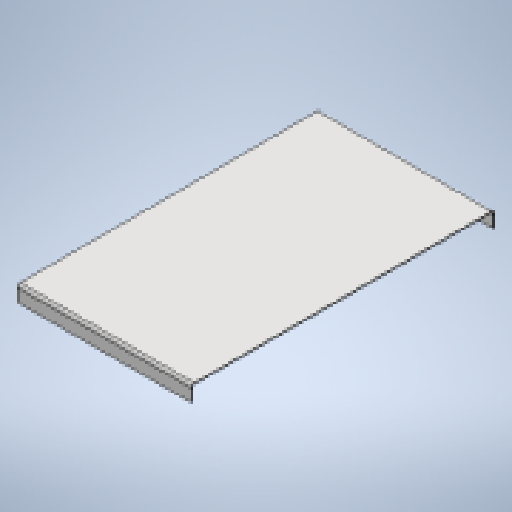
# Autodesk Inventor part: TRM 025 left board damper
Saved by Autodesk Inventor 2025 (Build 290162010, 162A)
## iProperties
Created: 2024-08-07
Part Number: TRM 025 left board damper
Material: AISI 304
Document SubType Name: Sheet Metal
Designer: pokla
Density: 8.02768 g/cm^3
Flat Pattern Width: 29 cm
Flat Pattern Length: 53.0404 cm
Flat Pattern Area: 1538.17 cm^2
Sheet Metal Rule: AISI304 2mm Die16
Sheet Metal Width: 290,000 mm
Sheet Metal Length: 530,404 mm
Sheet Metal Area: 153817,155 mm^2
Appearance: Default
Stock Number: ТРМ 025 левый борт успокоитель
Author: pokla
Autodesk Inventor part; units mm, degrees
ref_plane "YZ Plane" through (0, 0, 0) normal (1, 0, 0) x (0, 1, 0)
ref_plane "XZ Plane" through (0, 0, 0) normal (0, 1, 0) x (-1, 0, 0)
ref_plane "XY Plane" through (0, 0, 0) normal (0, 0, 1) x (1, 0, 0)
sketch "Sketch1" plane through (0, 0, 0) normal (0, 0, 1) x (1, 0, 0)
  line L0 (-145, -242) -> (145, -242)
  line L1 (145, -242) -> (145, 242)
  line L2 (145, 242) -> (-145, 242)
  line L3 (-145, 242) -> (-145, -242)
  line L4 (-145, -242) -> (145, 242) construction
  line L5 (145, -242) -> (-145, 242) construction
  point P0 (0, 0)
  dimension "d0" = 290
  dimension "d1" = 484
  measures "d0" distance of L2.end L1.end
  measures "d1" distance of L1.end L0.end
extrude "Plate1" add sketch "Sketch1" along normal blind 2
sketch "Sketch2" plane through (0, 0, 0) normal (0, 0, -1) x (-1, 0, 0)
  line L0 (-125, 222) -> (75, 222) construction
  line L1 (75, 222) -> (75, 202) construction
  line L2 (75, 202) -> (-125, 202) construction
  line L3 (-125, 202) -> (-125, 222) construction
  line L4 (-145, 242) -> (145, 242) projected
  line L5 (-145, -242) -> (-145, 242) projected
  point P0 (0, 0)
  point P1 (-48, 100)
  point P2 (-50, 98)
  dimension "d6" = 200
  dimension "d9" = 20
  dimension "d10" = 20
  dimension "d11" = 20
  constraints: 4 other
  measures "d6" distance of L0.start L0.end
  measures "d9" distance of L0.end L1.end
  measures "d11" length of L3
mark "Mark1"
sketch "Sketch3" plane through (-145, 244, 2) normal (0, -1, 0) x (1, 0, 0)
  line L0 (290, 0) -> (0, 0)
  line L1 (0, 0) -> (0, 25)
  line L2 (0, 25) -> (290, 25)
  line L3 (290, 25) -> (290, 0)
  constraints: 8 end point
edge flange "Flange1" height 25 angle 90 thickness 2 bend radius 2.75 thickness toward (0, -1, 0) relief round relief width 2 relief depth 1 corner gap 2.75 corner form 0 edges at (0, 242, 2) (0, -242, 2) wall of the first edge with corners at (145, 244, 2) (-145, 244, 2) (-145, 244, -23) (145, 244, -23)
bend "Bend1"
corner "Corner1"
equation "\"d2\" = Thickness"
equation "\"d12\" = BendReliefWidth"
equation "\"d13\" = BendReliefDepth"
equation "\"d14\" = MinimumRemnant"
equation "\"d15\" = TransitionRadius"
equation "\"d18\" = BendRadius"
equation "\"d19\" = CornerReliefSize"
equation "\"d20\" = GapSize"
equation "\"d21\" = JacobiRadiusSize"
equation "\"BendReliefWidth\" = Thickness"
equation "\"BendReliefDepth\" = 0.5 * Thickness"
equation "\"CornerReliefSize\" = 4 * Thickness"
equation "\"MinimumRemnant\" = 2 * Thickness"
equation "\"TransitionRadius\" = BendRadius"
equation "\"JacobiRadiusSize\" = BendRadius"
equation "\"GapSize\" = Thickness"
equation "\"Thickness\" = 2"
equation "\"BendRadius\" = 2.75"
body "Solid1"
